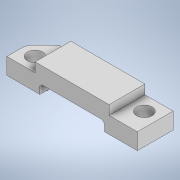
# Autodesk Inventor part: IMU_clamp
Saved by Autodesk Inventor 2022 (Build 260153000, 153)
## iProperties
Created: 2021-10-22
Part Number: IMU_clamp
Material: Generic
Document SubType Name: Modeling
Designer: kylem
Density: 1 g/cm^3
Appearance: Default
Author: kylem
Autodesk Inventor part; units mm, degrees
ref_plane "YZ Plane" through (0, 0, 0) normal (1, 0, 0) x (0, 1, 0)
ref_plane "XZ Plane" through (0, 0, 0) normal (0, 1, 0) x (-1, 0, 0)
ref_plane "XY Plane" through (0, 0, 0) normal (0, 0, 1) x (1, 0, 0)
sketch "Sketch1" plane through (0, 0, 0) normal (0, 1, 0) x (-1, 0, 0)
  line L0 (0, 0) -> (17.75, 0)
  line L1 (17.75, 0) -> (17.75, -7)
  line L2 (17.75, -7) -> (0, -7)
  line L3 (0, -7) -> (0, 0)
  dimension "d0" = 17.75
  dimension "d1" = 7
  constraints: 8 end point, 2 parallel, 1 horizontal, 1 perpendicular
  measures "d0" distance of L1.end L2.end
  measures "d1" distance of L0.end L1.end
extrude "Extrusion1" add sketch "Sketch1" along normal blind 2
sketch "Sketch2" plane through (0, 0, 0) normal (0, -1, 0) x (1, 0, 0)
  line L0 (-17.75, 0) -> (0, 0) projected
  line L1 (0, -7) -> (-17.75, -7) projected
  line L2 (0, 0) -> (-2, 0)
  line L3 (-2, 0) -> (-2, -7)
  line L4 (-2, -7) -> (0, -7)
  line L5 (0, -7) -> (0, 0)
  line L6 (-17.75, -7) -> (-17.75, 0) projected
  line L7 (-17.75, 0) -> (-15.75, 0)
  line L8 (-15.75, 0) -> (-15.75, -7)
  line L9 (-15.75, -7) -> (-17.75, -7)
  line L10 (-17.75, -7) -> (-17.75, 0)
  dimension "d4" = 2
  dimension "d5" = 2
  constraints: 16 end point, 4 parallel, 2 horizontal, 2 perpendicular, 2 point on line
  measures "d4" distance of L4.end L3.end
  measures "d5" distance of L8.end L9.end
extrude "Extrusion2" add sketch "Sketch2" along normal blind 2 contours L0 L8 L1 L6 | L0 L5 L1 L3
sketch "Sketch3" plane through (0, -2, 0) normal (0, -1, 0) x (1, 0, 0)
  line L0 (0, 0) -> (-1, 0)
  line L1 (0, 0) -> (-2, 0) projected
  line L2 (-1, 0) -> (-1, -2.334)
  line L3 (-1, 0) -> (-1, -4.915)
  circle A0 centre (-1, -2.334) radius 0.35
  circle A1 centre (-1, -4.915) radius 0.35
  line L4 (0, 0) -> (0, -7) projected
  line L5 (-17.75, -7) -> (-17.75, 0) projected
  line L6 (0, 0) -> (-17.75, 0)
  line L7 (-15.75, 0) -> (-2, 0) projected
  line L8 (-8.875, 0) -> (-8.875, -0.7455)
  circle A2 centre (-16.75, -2.334) radius 0.35
  circle A3 centre (-16.75, -4.915) radius 0.35
  dimension "d8" = 1
  dimension "d9" = 2.334
  dimension "d10" = 4.915
  dimension "d11" = 0.7
  dimension "d12" = 0.7
  constraints: 10 end point, 4 centre point, 2 coincident, 2 midpoint, 2 symmetric about line, 2 vertical, 1 horizontal, 1 perpendicular, 2 other
  measures "d8" distance of L0.start L0.end
  measures "d9" distance of L0.end L2.end
  measures "d10" distance of L0.end L3.end
  measures "d11" diameter of A0
  measures "d12" diameter of A1
extrude "Extrusion3" add sketch "Sketch3" along normal blind 0.8
sketch "Sketch4" plane through (0, 2, -7) normal (0, 0, -1) x (-1, 0, 0)
  line L0 (0, 0) -> (0, -4) projected
  line L1 (0, -4) -> (-4, -4)
  line L2 (-4, -4) -> (-4, -2)
  line L3 (-4, -2) -> (0, -2)
  line L4 (0, -2) -> (0, -4)
  line L5 (17.75, -4) -> (17.75, 0) projected
  line L6 (17.75, -4) -> (21.75, -4)
  line L7 (21.75, -4) -> (21.75, -2)
  line L8 (21.75, -2) -> (17.75, -2)
  line L9 (17.75, -2) -> (17.75, -4)
  dimension "d19" = 4
  dimension "d20" = 2
  dimension "d21" = 4
  dimension "d22" = 2
  constraints: 16 end point, 4 parallel, 2 horizontal, 2 perpendicular
  measures "d19" distance of L2.end L3.end
  measures "d20" distance of L1.end L2.end
  measures "d21" distance of L8.end L7.end
  measures "d22" distance of L7.end L6.end
extrude "Extrusion4" add sketch "Sketch4" against normal blind 7
sketch "Sketch6" plane through (0, 0, -7) normal (0, 1, 0) x (1, 0, 0)
  line L0 (0, -7) -> (0, 0) projected
  line L1 (4, 0) -> (4, -7) projected
  line L2 (0, -7) -> (4, -7)
  line L3 (4, -7) -> (4, 0)
  line L4 (4, 0) -> (0, 0)
  line L5 (0, 0) -> (0, -7)
  line L6 (-15.75, -7) -> (-21.75, -7) projected
  line L7 (0, 0) -> (-17.75, 0) projected
  line L8 (-21.75, -7) -> (-17.75, -7)
  line L9 (-17.75, -7) -> (-17.75, 0)
  line L10 (-17.75, 0) -> (-21.75, 0)
  line L11 (-21.75, 0) -> (-21.75, -7)
  constraints: 16 end point, 4 parallel, 2 horizontal, 2 perpendicular
extrude "Extrusion5" add sketch "Sketch6" along normal blind 2
sketch "Sketch8" plane through (0, 2, 0) normal (0, 1, 0) x (1, 0, 0)
  line L0 (4, 0) -> (4, 7) projected
  line L1 (4, 0) -> (5, 0)
  line L2 (5, 0) -> (5, 7)
  line L3 (5, 7) -> (4, 7)
  line L4 (4, 7) -> (4, 0)
  line L5 (-21.75, 7) -> (-21.75, 0) projected
  line L6 (-21.75, 0) -> (-22.75, 0)
  line L7 (-22.75, 0) -> (-22.75, 7)
  line L8 (-22.75, 7) -> (-21.75, 7)
  line L9 (-21.75, 7) -> (-21.75, 0)
  point P0 (0, 0)
  dimension "d33" = 1
  dimension "d34" = 1
  constraints: 16 end point, 4 parallel, 2 horizontal, 2 perpendicular, 1 point on line
  measures "d33" distance of L3.end L2.end
  measures "d34" distance of L7.end L8.end
extrude "Extrusion6" add sketch "Sketch8" against normal blind 4
sketch "Sketch9" plane through (0, 2, 0) normal (0, 1, 0) x (1, 0, 0)
  line L0 (-2, 0) -> (5, 0) projected
  line L1 (5, 0) -> (2, 0)
  line L2 (2, 0) -> (2, 4.5)
  line L3 (2, 4.5) -> (5, 4.5)
  line L4 (5, 4.5) -> (5, 0)
  line L5 (-22.75, 0) -> (5, 0) projected
  line L6 (-22.75, 0) -> (-19.75, 0)
  line L7 (-19.75, 0) -> (-19.75, 3)
  line L8 (-19.75, 3) -> (-22.75, 3)
  line L9 (-22.75, 3) -> (-22.75, 0)
  circle A0 centre (2, 4.5) radius 1.65
  circle A1 centre (-19.75, 3) radius 1.65
  point P0 (0, 0)
  dimension "d37" = 3
  dimension "d38" = 4.5
  dimension "d39" = 3
  dimension "d40" = 3
  dimension "d41" = 3.3
  dimension "d42" = 3.3
  constraints: 16 end point, 4 parallel, 2 centre point, 2 coincident, 2 horizontal, 2 perpendicular
  measures "d37" distance of L2.end L3.end
  measures "d38" distance of L1.end L2.end
  measures "d39" distance of L8.end L7.end
  measures "d40" distance of L7.end L6.end
  measures "d41" diameter of A0
  measures "d42" diameter of A1
extrude "Extrusion7" cut sketch "Sketch9" against normal blind 4 contours A0 L3 L2 | L2 L3 A0 | A1 L8 L7 | L7 L8 A1
sketch "Sketch10" plane through (0, 2, 0) normal (0, 1, 0) x (1, 0, 0)
  line L0 (9.5944, -4.5178) -> (-29.7564, -4.5178)
  line L1 (-29.7564, -4.5178) -> (-29.7564, 11.1864)
  line L2 (-29.7564, 11.1864) -> (9.5944, 11.1864)
  line L3 (9.5944, 11.1864) -> (9.5944, -4.5178)
  point P0 (0, 0)
  constraints: 8 end point, 2 parallel, 1 horizontal, 1 perpendicular
extrude "Extrusion8" cut sketch "Sketch10" against normal blind 0.5
sketch "Sketch11" plane through (0, 1.5, 0) normal (0, 1, 0) x (1, 0, 0)
  circle A0 centre (2, 4.5) radius 1.65 projected
  line L0 (2, 4.5) -> (-1, 4.5)
  circle A1 centre (-19.75, 3) radius 1.65 projected
  line L1 (-19.75, 3) -> (-16.75, 3)
  line L2 (-16.75, 3) -> (-16.75, 7.7148)
  line L3 (-22.75, 7) -> (5, 7) projected
  line L4 (5, 0) -> (-22.75, 0) projected
  line L5 (-16.75, 7) -> (-1, 7)
  line L6 (-1, 7) -> (-1, 0)
  line L7 (-1, 0) -> (-16.75, 0)
  line L8 (-16.75, 0) -> (-16.75, 7)
  point P0 (0, 0)
  point P1 (-16.75, 0)
  point P2 (-1, 7)
  dimension "d47" = 3
  dimension "d48" = 3
  constraints: 14 end point, 3 horizontal, 3 point on line, 2 parallel, 2 perpendicular
  measures "d47" distance of L0.start L0.end
  measures "d48" distance of L1.start L1.end
extrude "Extrusion9" add sketch "Sketch11" along normal blind 2 contours L2 L3 L6 L4 L8
chamfer "Chamfer1" distance 0.5 angle 45 2 edges at (-2, 0, -3.5) (-15.75, 0, -3.5)
sketch "Sketch12" plane through (0, -2, 0) normal (0, -1, 0) x (1, 0, 0)
  line L0 (-15.75, 0) -> (-15.75, -7) projected
  line L1 (-15.75, -7) -> (-22.75, -7) projected
  line L2 (-15.75, 0) -> (-17.75, 0)
  line L3 (-17.75, 0) -> (-17.75, -7)
  line L4 (-17.75, -7) -> (-15.75, -7)
  line L5 (-15.75, -7) -> (-15.75, 0)
  line L6 (-22.75, 0) -> (-22.75, -7) projected
  line L7 (-17.75, -7) -> (-22.75, -7)
  line L8 (-22.75, -7) -> (-22.75, 0)
  line L9 (-22.75, 0) -> (-17.75, 0)
  line L10 (-17.75, 0) -> (-17.75, -7)
  point P0 (0, 0)
  dimension "d57" = 2
  constraints: 16 end point, 4 parallel, 2 horizontal, 2 perpendicular, 1 point on line
  measures "d57" distance of L4.end L3.end
sketch "Sketch13" plane through (-15.75, -2, -7) normal (0, 0, -1) x (-1, 0, 0)
  line L0 (0, 0) -> (7, 0) projected
  line L1 (1, 3.5) -> (7, 3.5) projected
  line L2 (0, 0) -> (7, 0)
  line L3 (7, 0) -> (7, 3.5)
  line L4 (7, 3.5) -> (0, 3.5)
  line L5 (0, 1.5) -> (0, 0)
  line L6 (-13.75, 0) -> (-20.75, 0) projected
  line L7 (-20.75, 3.5) -> (-20.75, 0) projected
  line L8 (-13.75, 0) -> (-20.75, 0)
  line L9 (-20.75, 0) -> (-20.75, 3.5)
  line L10 (-20.75, 3.5) -> (-13.75, 3.5)
  line L11 (-14.75, 5.5) -> (1, 5.5) projected
  line L12 (-14.75, 5.5) -> (1, 5.5)
  line L13 (1, 5.5) -> (1, 2)
  line L14 (-14.75, 2) -> (-14.75, 5.5)
  line L15 (0, 1.5) -> (-0.5, 2) projected
  line L16 (0, 1.5) -> (-0.5, 2)
  line L17 (-13.75, 1.5) -> (-13.75, 0) projected
  line L18 (-13.25, 2) -> (-13.75, 1.5) projected
  line L19 (-13.75, 1.5) -> (-13.25, 2)
  line L20 (-13.75, 1.5) -> (-13.75, 0)
  line L21 (-0.5, 2) -> (-13.25, 2)
  point P0 (-15.75, 2)
  point P1 (-14.75, 3.5)
  constraints: 28 end point, 6 parallel, 3 horizontal, 3 perpendicular, 2 collinear, 1 point on line
extrude "Extrusion10" add sketch "Sketch13" along normal blind 0.6
chamfer "Chamfer3" distance 3.5 angle 45 1 edges at (-22.75, -0.25, -7.6)
chamfer "Chamfer4" distance 0.5 angle 45 1 edges at (-21, -2, -5.85)
chamfer "Chamfer5" distance 0.5 angle 45 1 edges at (-22.75, 0, -4.1)
body "Solid1"
